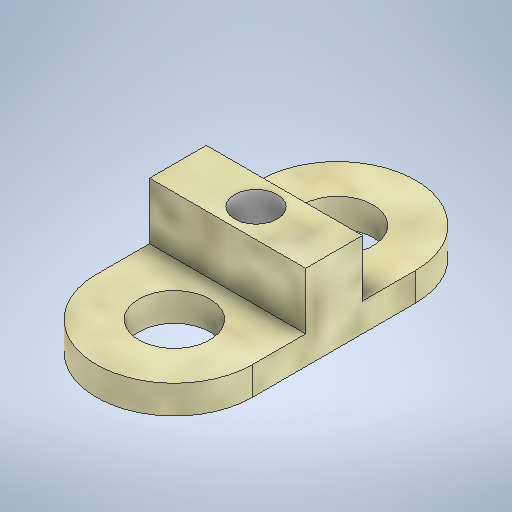
# Autodesk Inventor part: bearing plate
Saved by Autodesk Inventor 2025.1 (Build 291241000, 241)
## iProperties
Created: 2024-10-07
Part Number: bearing plate
Material: Generic
Document SubType Name: Modeling
Designer: m_kni
Density: 1 g/cm^3
Appearance: Default
Author: m_kni
Autodesk Inventor part; units mm, degrees
ref_plane "YZ Plane" through (0, 0, 0) normal (1, 0, 0) x (0, 1, 0)
ref_plane "XZ Plane" through (0, 0, 0) normal (0, 1, 0) x (-1, 0, 0)
ref_plane "XY Plane" through (0, 0, 0) normal (0, 0, 1) x (1, 0, 0)
sketch "Sketch1" plane through (0, 0, 0) normal (0, 1, 0) x (-1, 0, 0)
  circle A0 centre (0, 11.1484) radius 5.5
  line L0 (0, 11.1484) -> (0, -0.3516)
  circle A1 centre (0, -0.3516) radius 5.5
  circle A2 centre (0, 11.1484) radius 2.5
  circle A3 centre (0, -0.3516) radius 2.5
  line L1 (5.5, 11.1484) -> (5.5, -0.3516)
  line L2 (-5.5, 11.1484) -> (-5.5, -0.3516)
  point P0 (0, 0)
  dimension "d0" = 11
  dimension "d1" = 11.5
  dimension "d2" = 11
  dimension "d3" = 5
  dimension "d4" = 5
  constraints: 6 end point, 4 centre point, 4 point on circle, 3 coincident, 2 tangent, 1 vertical
  measures "d0" diameter of A0
  measures "d1" distance of L0.start L0.end
  measures "d2" diameter of A1
  measures "d3" diameter of A2
  measures "d4" diameter of A3
extrude "Extrusion1" add sketch "Sketch1" along normal blind 2
sketch "Sketch2" plane through (0, 2, 0) normal (0, 1, 0) x (1, 0, 0)
  circle A0 centre (0, -11.1484) radius 2.5 projected
  line L0 (0, -8.6484) -> (0, -2.1484)
  circle A1 centre (0, 0.3516) radius 2.5 projected
  line L1 (-5.5, 0.3516) -> (-5.5, -11.1484) projected
  line L2 (5.5, -3.3984) -> (-5.5, -3.3984)
  line L3 (-5.5, -3.3984) -> (-5.5, -7.3984)
  line L4 (-5.5, -7.3984) -> (5.5, -7.3984)
  line L5 (5.5, -7.3984) -> (5.5, -3.3984)
  line L6 (5.5, -3.3984) -> (-5.5, -7.3984) construction
  line L7 (-5.5, -3.3984) -> (5.5, -7.3984) construction
  point P0 (0, 0)
  point P1 (0, -5.3984)
  dimension "d7" = 4
  constraints: 14 end point, 3 midpoint, 2 parallel, 2 vertical alignment, 1 horizontal, 1 perpendicular, 1 point on line, 1 vertical, 2 other
  measures "d7" distance of L3.end L2.end
extrude "Extrusion2" add sketch "Sketch2" along normal blind 4 contours L4 L1 L2 L0 | L0 L2 L5 L4
sketch "Sketch3" plane through (0, 6, 0) normal (0, 1, 0) x (1, 0, 0)
  line L0 (5.5, -3.3984) -> (-5.5, -3.3984) projected
  line L1 (-5.5, -3.3984) -> (-5.5, -7.3984) projected
  line L2 (-5.5, -7.3984) -> (5.5, -7.3984) projected
  line L3 (5.5, -7.3984) -> (5.5, -3.3984) projected
  circle A0 centre (0, -5.3984) radius 1.5
  point P0 (0, 0)
  dimension "d14" = 3
  constraints: 1 centre point
  measures "d14" diameter of A0
extrude "Extrusion3" cut sketch "Sketch3" against normal blind 16.6375 contours A0
body "Solid1"
